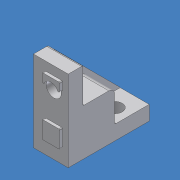
# Autodesk Inventor part: HBLFSL5hblfsn5
Saved by Autodesk Inventor 2014 SP1 (Build 180222100, 222)
## iProperties
Category: PARTsolutions
Created: 2015-02-04
Part Number: HBLFSL5hblfsn5
Catalog Web Link: www.cadenas.de
Description: HBLFSN5, HBLFSNB5, HBLFSNM5, HBLFSNK5, HBLFSSW5, HBLFSSWB5, HBLFSDW5 - Thin Reversal Brackets for Slot Width 6 Frames - For 20, 40mm Sections
Document SubType Name: Modeling
Designer: PARTsolutions
Material: Generic
Density: 1 g/cm^3
Appearance: RGB(192,192,192)
NB: HBLFSL5hblfsn5
NN: HBLFSN5, HBLFSNB5, HBLFSNM5, HBLFSNK5, HBLFSSW5, HBLFSSWB5, HBLFSDW5
NT: Thin Reversal Brackets for Slot Width 6 Frames - For 20, 40mm Sections
NBSYN: $PN.hblfsn5
LINA: HBLFSL5hblfsn5
PN: HBLFSL5
TP: HBLFSL5
NOH: 1
NOHV: 1
MAT: JIS-ADC12
ST: -
TYPE: HBLFSL5
FEAT: One Side Rib Bracket
MASS: 13
AB: CBM5-10
NOB: 2
AN: HNTT5-5
NON: 2
AL: 1176
W: 12
H: 28
DP: 28
T: 5.0
HDIS: 0
DPOS: 12.000
HH1: 21
BOLTX: 21.0
HV1: 21
BOLTY: 21.0
DIA: 5.2
ALT1OPT: '','w/o C (Mounting Holes for Cover)','-C','with C (Mounting Holes for Cover)'
ALT2OPT: '' , 'w/o Set Applicable Bolt & Nut' , '-SET' , 'with SET (Set Applicable Bolt & Nut)' , '-SST' , 'with SST (Stainless Steel Set Applicable Bolt & Nut)' , '-SEP' , 'with SEP (Post Assembly Spring Nuts Set Applicable Bolt & Nut)' , '-SSP' , 'with SSP (Post Assembly Spring Nuts, Stainless Steel Set Applicable Bolt & Nut)'
R: 1.000
R1: 0.300
APOSV: 0
VER: 2
PR: 4
TT: 1.0
T1: 0
KT: 4
SUPPLIER: Misumi
ARTICLENO: HBLFSL5hblfsn5
BOMINFO: HBLFSL5hblfsn5
CREATOR: CADENAS GmbH
PSOL_IDENT_0: {\\10.0.0.236\data_v8\23d-libs\misumi\metric\38_al_extrusions_blackets\5\hblfsn5.prj},242 {VTYP=3D},
PSOL_IDENT_1: {NB=HBLFSL5hblfsn5},{LINA=HBLFSL5hblfsn5},{NN=HBLFSN5, HBLFSNB5, HBLFSNM5, HBLFSNK5, HBLFSSW5, HBLFS
PSOL_IDENT_2: SWB5, HBLFSDW5},{DATE=19.11.2014 02:27:22},{GEOMDATE=28.01.2010 06:29:00},{VERSION=},{LINEID=240},{L
PSOL_IDENT_3: INESUBID=-1},{WBVAR=ALT1,ALT2}  {NB=HBLFSL5hblfsn5},{LINA=HBLFSL5hblfsn5},{KT=4},{PN=HBLFSL5},{TP=HB
PSOL_IDENT_4: LFSL5},{NOH=1},{NOHV=1},{MAT=JIS-ADC12},{ST=-},{TYPE=HBLFSL5},{FEAT=One Side Rib Bracket},{ALT1=},{A
PSOL_IDENT_5: LT2=},{MASS=13},{AB=CBM5-10},{NOB=2},{AN=HNTT5-5},{NON=2},{AL=1176},{W=12},{H=28},{DP=28},{T=5.0},{H
PSOL_IDENT_6: DIS=0},{DPOS=12},{HH1=21},{BOLTX=21.0},{HV1=21},{BOLTY=21.0},{DIA=5.2},{ALT1OPT='','w/o C (Mounting
PSOL_IDENT_7: Holes for Cover)','-C','with C (Mounting Holes for Cover)'},{ALT2OPT= '' , 'w/o Set Applicable Bolt
PSOL_IDENT_8: & Nut' , '-SET' , 'with SET (Set Applicable Bolt & Nut)' , '-SST' , 'with SST (Stainless Steel Set A
PSOL_IDENT_9: pplicable Bolt & Nut)' , '-SEP' , 'with SEP (Post Assembly Spring Nuts Set Applicable Bolt & Nut)' ,
PSOL_IDENT_10: '-SSP' , 'with SSP (Post Assembly Spring Nuts, Stainless Steel Set Applicable Bolt & Nut)' },{R=1},
PSOL_IDENT_11: {R1=0.3},{APOSV=0},{VER=2},{PR=4},{TT=1.0},{T1=0}
Title: HBLFSL5hblfsn5
Author: Cadenas PARTsolutions
Comments: Thin Reversal Brackets for Slot Width 6 Frames - For 20, 40mm Sections
Autodesk Inventor part; units mm, degrees
sketch "Sketch_15" plane through (0, 0, 0) normal (1, 0, 0) x (0, 1, 0)
  line L0 (0, 28) -> (0, 0)
  line L1 (0, 0) -> (28, 0)
  line L2 (28, 0) -> (28, 4.5858)
  arc A0 (28, 4.5858) -> (27.7071, 5.2929) centre (27, 4.5858) ccw
  line L3 (27.7071, 5.2929) -> (5.2929, 27.7071)
  arc A1 (5.2929, 27.7071) -> (4.5858, 28) centre (4.5858, 27) ccw
  line L4 (4.5858, 28) -> (0, 28)
  constraints: 10 end point, 4 point on circle, 2 centre point
extrude "Extrusion1" add sketch "Sketch_15" along normal mid plane 12
sketch "Sketch_60" plane through (0, -1, 0) normal (0, 1, 0) x (1, 0, 0)
  line L0 (-6, 0) -> (-6, -28)
  line L1 (-6, -28) -> (6, -28)
  line L2 (6, -28) -> (6, 0)
  line L3 (6, 0) -> (-6, 0)
  constraints: 8 end point
extrude "Extrusion2" add sketch "Sketch_60" along normal blind 1
sketch "Sketch_61" plane through (0, -1, 0) normal (0, 1, 0) x (1, 0, 0)
  line L0 (-6, 0) -> (-6, -28)
  line L1 (-6, -28) -> (6, -28)
  line L2 (6, -28) -> (6, 0)
  line L3 (6, 0) -> (-6, 0)
  arc A0 (-2, -10.7) -> (-1.7, -11) centre (-1.7, -10.7) ccw
  line L4 (-1.7, -11) -> (3.7, -11)
  arc A1 (3.7, -11) -> (4, -10.7) centre (3.7, -10.7) ccw
  line L5 (4, -10.7) -> (4, -5.3)
  arc A2 (4, -5.3) -> (3.7, -5) centre (3.7, -5.3) ccw
  line L6 (3.7, -5) -> (-1.7, -5)
  arc A3 (-1.7, -5) -> (-2, -5.3) centre (-1.7, -5.3) ccw
  line L7 (-2, -5.3) -> (-2, -10.7)
  arc A4 (-2, -24.7) -> (-1.7, -25) centre (-1.7, -24.7) ccw
  line L8 (-1.7, -25) -> (3.7, -25)
  arc A5 (3.7, -25) -> (4, -24.7) centre (3.7, -24.7) ccw
  line L9 (4, -24.7) -> (4, -22.3)
  arc A6 (4, -22.3) -> (3.7, -22) centre (3.7, -22.3) ccw
  line L10 (3.7, -22) -> (-1.7, -22)
  arc A7 (-1.7, -22) -> (-2, -22.3) centre (-1.7, -22.3) ccw
  line L11 (-2, -22.3) -> (-2, -24.7)
  constraints: 24 end point, 16 point on circle, 8 centre point
extrude "Extrusion3" cut sketch "Sketch_61" along normal blind 1
sketch "Sketch_62" plane through (0, 0, 0) normal (0, 0, 1) x (1, 0, 0)
  line L0 (-6, 0) -> (6, 0)
  line L1 (6, 0) -> (6, 28)
  line L2 (6, 28) -> (-6, 28)
  line L3 (-6, 28) -> (-6, 0)
  constraints: 8 end point
extrude "Extrusion4" add sketch "Sketch_62" along normal mid plane 2
sketch "Sketch_63" plane through (0, 0, -1) normal (0, 0, 1) x (1, 0, 0)
  line L0 (-6, 0) -> (6, 0)
  line L1 (6, 0) -> (6, 28)
  line L2 (6, 28) -> (-6, 28)
  line L3 (-6, 28) -> (-6, 0)
  line L4 (-2, 10.7) -> (-2, 5.3)
  arc A0 (-2, 5.3) -> (-1.7, 5) centre (-1.7, 5.3) ccw
  line L5 (-1.7, 5) -> (3.7, 5)
  arc A1 (3.7, 5) -> (4, 5.3) centre (3.7, 5.3) ccw
  line L6 (4, 5.3) -> (4, 10.7)
  arc A2 (4, 10.7) -> (3.7, 11) centre (3.7, 10.7) ccw
  line L7 (3.7, 11) -> (-1.7, 11)
  arc A3 (-1.7, 11) -> (-2, 10.7) centre (-1.7, 10.7) ccw
  line L8 (-2, 24.7) -> (-2, 22.3)
  arc A4 (-2, 22.3) -> (-1.7, 22) centre (-1.7, 22.3) ccw
  line L9 (-1.7, 22) -> (3.7, 22)
  arc A5 (3.7, 22) -> (4, 22.3) centre (3.7, 22.3) ccw
  line L10 (4, 22.3) -> (4, 24.7)
  arc A6 (4, 24.7) -> (3.7, 25) centre (3.7, 24.7) ccw
  line L11 (3.7, 25) -> (-1.7, 25)
  arc A7 (-1.7, 25) -> (-2, 24.7) centre (-1.7, 24.7) ccw
  constraints: 24 end point, 16 point on circle, 8 centre point
extrude "Extrusion5" cut sketch "Sketch_63" along normal blind 1
sketch "Sketch_12" plane through (-4, 0, 0) normal (1, 0, 0) x (0, 0, -1)
  line L0 (-28, 5) -> (-16.5, 5)
  arc A0 (-16.5, 5) -> (-16, 5.5) centre (-16.5, 5.5) ccw
  line L1 (-16, 5.5) -> (-16, 14)
  arc A1 (-14, 16) -> (-16, 14) centre (-14, 14) ccw
  line L2 (-14, 16) -> (-5.5, 16)
  arc A2 (-5.5, 16) -> (-5, 16.5) centre (-5.5, 16.5) ccw
  line L3 (-5, 16.5) -> (-5, 28)
  line L4 (-5, 28) -> (-28, 28)
  line L5 (-28, 28) -> (-28, 5)
  constraints: 12 end point, 6 point on circle, 3 centre point
extrude "Extrusion6" cut sketch "Sketch_12" along normal blind 16
sketch "Sketch_20" plane through (0, 0, 0) normal (0, 0, 1) x (1, 0, 0)
  circle A0 centre (1, 21) radius 2.6
  constraints: 1 centre point
extrude "Extrusion7" cut sketch "Sketch_20" along normal mid plane 10
sketch "Sketch_29" plane through (0, 0, 0) normal (0, 1, 0) x (-1, 0, 0)
  circle A0 centre (-1, 21) radius 2.6
  constraints: 1 centre point
extrude "Extrusion8" cut sketch "Sketch_29" along normal mid plane 10
ref_plane "to_bolt_row_1_to_3_XY" through (1, 21, 5) normal (0, 0, 1) x (1, 0, 0)
ref_plane "to_bolt_row_1_to_3_YZ" through (1, 21, 5) normal (1, 0, 0) x (0, 1, 0)
ref_plane "to_bolt_row_1_to_3_ZX" through (1, 21, 5) normal (0, 1, 0) x (0, 0, 1)
ref_plane "to_bolt_row_1_to_3_base_XY" through (1, 5, 21) normal (0, 1, 0) x (1, 0, 0)
ref_plane "to_bolt_row_1_to_3_base_YZ" through (1, 5, 21) normal (1, 0, 0) x (0, 0, -1)
ref_plane "to_bolt_row_1_to_3_base_ZX" through (1, 5, 21) normal (0, 0, -1) x (0, 1, 0)
ref_plane "to_nut_row_1_to_3_XY" through (1, 21, -2) normal (0, 0, 1) x (1, 0, 0)
ref_plane "to_nut_row_1_to_3_YZ" through (1, 21, -2) normal (1, 0, 0) x (0, 1, 0)
ref_plane "to_nut_row_1_to_3_ZX" through (1, 21, -2) normal (0, 1, 0) x (0, 0, 1)
ref_plane "to_nut_row_1_to_3_base_XY" through (1, -2, 21) normal (0, 1, 0) x (1, 0, 0)
ref_plane "to_nut_row_1_to_3_base_YZ" through (1, -2, 21) normal (1, 0, 0) x (0, 0, -1)
ref_plane "to_nut_row_1_to_3_base_ZX" through (1, -2, 21) normal (0, 0, -1) x (0, 1, 0)
ref_plane "bracket_to_dummy_XY" through (0, 0, 0) normal (0, 1, 0) x (1, 0, 0)
ref_plane "bracket_to_dummy_YZ" through (0, 0, 0) normal (1, 0, 0) x (0, 0, -1)
ref_plane "bracket_to_dummy_ZX" through (0, 0, 0) normal (0, 0, -1) x (0, 1, 0)
ref_plane "bracket_to_bolt_XY" through (1, 21, 0) normal (0, 0, 1) x (1, 0, 0)
ref_plane "bracket_to_bolt_YZ" through (1, 21, 0) normal (1, 0, 0) x (0, 1, 0)
ref_plane "bracket_to_bolt_ZX" through (1, 21, 0) normal (0, 1, 0) x (0, 0, 1)
body "Solid1"
